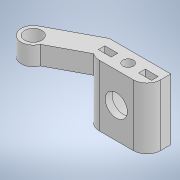
# Autodesk Inventor part: Деталь крепления диска к поворотному механизму
Saved by Autodesk Inventor 2020 (Build 240168000, 168)
## iProperties
Created: 2021-03-15
Part Number: Деталь крепления диска к поворотному механизму
Material: Типовые
Document SubType Name: Modeling
Designer: Антон
Density: 1 g/cm^3
Appearance: По умолчанию
Mass: 2.90777 g
Surface Area: 27.0682 cm^2
Volume: 2.90777 cm^3
Угол_Аккермана: 18,14 град
Высота_сошки: 21,000 мм
Ширина_колесной_базы: 59,900 мм
Длина_колесной_базы: 91,400 мм
Author: Антон
Autodesk Inventor part; units mm, degrees
ref_plane "YZ Plane" through (0, 0, 0) normal (1, 0, 0) x (0, 1, 0)
ref_plane "XZ Plane" through (0, 0, 0) normal (0, 1, 0) x (-1, 0, 0)
ref_plane "XY Plane" through (0, 0, 0) normal (0, 0, 1) x (1, 0, 0)
sketch "Эскиз1" plane through (0, 0, 0) normal (0, 0, 1) x (1, 0, 0)
  line L0 (0, 0) -> (18, 0)
  line L1 (18, 0) -> (18, 18)
  line L2 (18, 18) -> (0, 18)
  line L3 (0, 18) -> (0, 0)
  dimension "d0" = 18
  dimension "d1" = 18
  constraints: 8 end point, 2 parallel, 1 horizontal, 1 perpendicular
  measures "d0" distance of L2.end L1.end
  measures "d1" distance of L1.end L0.end
extrude "Выдавливание1" add sketch "Эскиз1" along normal blind 7
sketch "Эскиз2" plane through (0, 0, 0) normal (0, 0, -1) x (-1, 0, 0)
  line L0 (0, 0) -> (-18, 0) projected
  line L1 (-9, 0) -> (-9, 18)
  line L2 (-18, 18) -> (0, 18) projected
  circle A0 centre (-9, 9) radius 4.05
  dimension "d4" = 8.1
  constraints: 3 midpoint, 2 end point, 1 centre point
  measures "d4" diameter of A0
extrude "Выдавливание2" cut sketch "Эскиз2" against normal blind 5
sketch "Эскиз5" plane through (0, 18, 0) normal (0, 1, 0) x (1, 0, 0)
  line L0 (0, 0) -> (18, 0) projected
  line L1 (9, 0) -> (9, -3.5)
  circle A0 centre (9, -3.5) radius 1.55
  dimension "d21" = 3.5
  dimension "d22" = 3.1
  constraints: 2 end point, 1 centre point, 1 coincident, 1 midpoint, 1 vertical
  measures "d21" distance of L1.start L1.end
  measures "d22" diameter of A0
extrude "Выдавливание4" cut sketch "Эскиз5" against normal blind 4
sketch "Эскиз6" plane through (0, 0, 0) normal (0, -1, 0) x (1, 0, 0)
  circle A0 centre (9, 3.5) radius 1.55 projected
  point P0 (0, 0)
  point P1 (7.5329, 7)
  point P2 (10.4671, 7)
  constraints: 1 other
extrude "Выдавливание5" cut sketch "Эскиз6" against normal blind 4
sketch "Эскиз8" plane through (0, 0, 7) normal (0, 0, 1) x (1, 0, 0)
  circle A0 centre (9, 9) radius 4.05 projected
  circle A1 centre (9, 9) radius 4.05 projected
  circle A2 centre (9, 9) radius 3.25
  point P0 (0, 0)
  dimension "d27" = 6.5
  constraints: 1 centre point, 1 coincident
  measures "d27" diameter of A2
extrude "Выдавливание6" cut sketch "Эскиз8" against normal through all contours A2
sketch "Эскиз22" plane through (0, 0, 0) normal (0, 0, -1) x (-1, 0, 0)
  circle A0 centre (-9, 9) radius 4.05 projected
  line L0 (0, 0) -> (-18, 0) projected
  line L1 (0, 18) -> (0, 0) projected
  line L2 (-18, 18) -> (0, 18) projected
  line L3 (-18, 0) -> (-18, 18) projected
  line L4 (-18, 18) -> (-11.8638, 11.8638) construction
  line L5 (0, 18) -> (-6.1362, 11.8638) construction
  line L6 (-18, 0) -> (-11.8638, 6.1362) construction
  line L7 (0, 0) -> (-18, 0) construction
  line L8 (0, 0) -> (-6.1362, 6.1362) construction
  point P0 (-14.9319, 14.9319)
  point P1 (-3.0681, 14.9319)
  point P2 (-3.0681, 3.0681)
  point P3 (-14.9319, 3.0681)
  constraints: 8 end point, 4 midpoint, 4 point on circle, 2 collinear
hole "Отверстие4" at (14.9319, 14.9319, 0) at (3.0681, 14.9319, 0) at (14.9319, 3.0681, 0) at (3.0681, 3.0681, 0) direction (0, 0, 1) diameter 2.2 depth 2.525
sketch "Эскиз23" plane through (0, 0, 0) normal (0, 0, -1) x (-1, 0, 0)
  circle A0 centre (-14.9319, 14.9319) radius 1.1 projected
  line L0 (-16.8319, 16.0289) -> (-14.9319, 17.1258)
  line L1 (-14.9319, 17.1258) -> (-13.0319, 16.0289)
  line L2 (-13.0319, 16.0289) -> (-13.0319, 13.8349)
  line L3 (-13.0319, 13.8349) -> (-14.9319, 12.738)
  line L4 (-14.9319, 12.738) -> (-16.8319, 13.8349)
  line L5 (-16.8319, 13.8349) -> (-16.8319, 16.0289)
  circle A1 centre (-3.0681, 14.9319) radius 1.1 projected
  line L6 (-1.1681, 13.8349) -> (-3.0681, 12.738)
  line L7 (-3.0681, 12.738) -> (-4.9681, 13.8349)
  line L8 (-4.9681, 13.8349) -> (-4.9681, 16.0289)
  line L9 (-4.9681, 16.0289) -> (-3.0681, 17.1258)
  line L10 (-3.0681, 17.1258) -> (-1.1681, 16.0289)
  line L11 (-1.1681, 16.0289) -> (-1.1681, 13.8349)
  circle A2 centre (-14.9319, 3.0681) radius 1.1 projected
  line L12 (-14.9319, 0.8742) -> (-16.8319, 1.9711)
  line L13 (-16.8319, 1.9711) -> (-16.8319, 4.1651)
  line L14 (-16.8319, 4.1651) -> (-14.9319, 5.262)
  line L15 (-14.9319, 5.262) -> (-13.0319, 4.1651)
  line L16 (-13.0319, 4.1651) -> (-13.0319, 1.9711)
  line L17 (-13.0319, 1.9711) -> (-14.9319, 0.8742)
  circle A3 centre (-3.0681, 3.0681) radius 1.1 projected
  line L18 (-4.9681, 1.9711) -> (-4.9681, 4.1651)
  line L19 (-4.9681, 4.1651) -> (-3.0681, 5.262)
  line L20 (-3.0681, 5.262) -> (-1.1681, 4.1651)
  line L21 (-1.1681, 4.1651) -> (-1.1681, 1.9711)
  line L22 (-1.1681, 1.9711) -> (-3.0681, 0.8742)
  line L23 (-3.0681, 0.8742) -> (-4.9681, 1.9711)
  line L24 (0, 0) -> (-18, 0) projected
  line L25 (-18, 18) -> (0, 18) projected
  line L26 (-18, 0) -> (-18, 18) projected
  line L27 (0, 18) -> (0, 0) projected
  line L28 (-16.8319, 1.9711) -> (-13.0319, 1.9711)
  line L29 (-13.0319, 1.9711) -> (-13.0319, 0)
  line L30 (-13.0319, 0) -> (-16.8319, 0)
  line L31 (-16.8319, 0) -> (-16.8319, 1.9711)
  line L32 (-4.9681, 1.9711) -> (-1.1681, 1.9711)
  line L33 (-1.1681, 1.9711) -> (-1.1681, 0)
  line L34 (-1.1681, 0) -> (-4.9681, 0)
  line L35 (-4.9681, 0) -> (-4.9681, 1.9711)
  line L36 (-4.9681, 16.0289) -> (-1.1681, 16.0289)
  line L37 (-1.1681, 16.0289) -> (-1.1681, 18)
  line L38 (-1.1681, 18) -> (-4.9681, 18)
  line L39 (-4.9681, 18) -> (-4.9681, 16.0289)
  line L40 (-16.8319, 16.0289) -> (-13.0319, 16.0289)
  line L41 (-13.0319, 16.0289) -> (-13.0319, 18)
  line L42 (-13.0319, 18) -> (-16.8319, 18)
  line L43 (-16.8319, 18) -> (-16.8319, 16.0289)
  point P0 (-14.8502, 16.0289)
  point P1 (-15.0135, 16.0289)
  point P2 (-1.1681, 0)
  dimension "d92" = 3.8
  constraints: 80 end point, 12 parallel, 4 coincident, 4 horizontal, 4 perpendicular, 3 collinear, 3 equal length, 3 point on line, 52 other
  measures "d92" distance between parallel lines of L8 L11
extrude "Выдавливание13" cut sketch "Эскиз23" against normal blind 1.95 from surface at -2.525 contours A0 L40 | A0 L40 L2 L3 L4 L5 | L40 A0 | A0 L40 L0 L1 | L1 L0 L43 L25 L41 | L25 L37 L10 L9 L39 | L36 A1 L11 L6 L7 L8 | L9 L10 L36 A1 | L36 A1 | A1 L36 | L31 L12 L17 L29 L24 | L28 A2 L17 L12 | L13 L14 L15 L16 L28 A2 | L24 L35 L23 L22 L33 | L28 A2 | A2 L28 | L32 A3 L18 L19 L20 L21 | L22 L23 L32 A3 | L32 A3 | A3 L32
sketch "Эскиз24" plane through (0, 18, 0) normal (0, 1, 0) x (1, 0, 0)
  circle A0 centre (9, -3.5) radius 1.55 projected
  circle A1 centre (9, -3.5) radius 1.55 projected
  line L0 (9, -3.5) -> (-12, -10.3813) construction
  line L1 (18, 0) -> (0, 0) projected
  circle A2 centre (-12, -10.3813) radius 2.525
  line L2 (0, 0) -> (0, -7) projected
  line L3 (18, -7) -> (0, -7) projected
  line L4 (-13.6564, -7.2697) -> (0, 0)
  line L5 (0, -7) -> (-8.7051, -11.634)
  circle A3 centre (-12, -10.3813) radius 3.525
  dimension "Угол_Аккермана" = 18.143
  dimension "d96" = 5.05
  dimension "Высота_сошки" = 21
  dimension "d116" = 7.05
  constraints: 6 end point, 2 centre point, 2 coincident, 2 point on circle, 1 parallel, 1 tangent
  measures "Угол_Аккермана" angle of L1 L0
  measures "d96" diameter of A2
  measures "Высота_сошки" horizontal distance of A0.centre L0.end
  measures "d116" diameter of A3
extrude "Выдавливание14" add sketch "Эскиз24" against normal blind 4 contours L2 L5 A3 L4 | A3
sketch "Эскиз26" plane through (0, 14, 0) normal (0, -1, 0) x (1, 0, 0)
  line L0 (0, 7) -> (-8.7051, 11.634) projected
  arc A0 (-8.7051, 11.634) -> (-13.6564, 7.2697) centre (-12, 10.3813) ccw projected
  line L1 (-13.6564, 7.2697) -> (0, 0) projected
  line L2 (0, 7) -> (0, 0) projected
  circle A1 centre (-12, 10.3813) radius 2.525 projected
  point P0 (0, 0)
extrude "Выдавливание16" add sketch "Эскиз26" along normal blind 1.5 contours L2 L1 A0 L0 | A1
fillet "Сопряжение13" radius 4 4 edges at (18, 9, 7) (0, 6.25, 7) (0, 13.25, 7) (0, 16, 7)
equation "\"Ширина_колесной_базы\" = 59.9"
equation "\"Длина_колесной_базы\" = 91.4"
